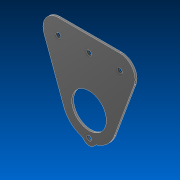
# Autodesk Inventor part: Intake Motor Holder Using 1__16 Gray Tinted Polycarbonate Sheet (36 x 72) (217-6627)
Saved by Autodesk Inventor 2022.2 (Build 262287000, 287)
## iProperties
Created: 2022-01-11
Part Number: Intake Motor Holder Using 1__16 Gray Tinted Polycarbonate Sheet (36 x 72) (217-6627)
Material: Polycarbonate, Clear
Document SubType Name: Modeling
Designer: omard
Density: 1.2 g/cm^3
Appearance: Smooth - Black
Author: omard
Autodesk Inventor part; units mm, degrees
ref_plane "YZ Plane" through (0, 0, 0) normal (1, 0, 0) x (0, 1, 0)
ref_plane "XZ Plane" through (0, 0, 0) normal (0, 1, 0) x (-1, 0, 0)
ref_plane "XY Plane" through (0, 0, 0) normal (0, 0, 1) x (1, 0, 0)
sketch "Sketch1" plane through (0, 0, 0) normal (0, 0, 1) x (1, 0, 0)
  circle A0 centre (0, 0) radius 14.2875
  circle A1 centre (-25.4, 41.275) radius 2.0701
  circle A2 centre (0, 41.275) radius 2.0701
  circle A3 centre (25.4, 41.275) radius 2.0701
  line L0 (-25.4, 41.275) -> (25.4, 41.275) construction
  circle A4 centre (0, 0) radius 22.225
  line L1 (-25.4, 41.275) -> (25.4, 41.275) construction
  line L2 (-25.4, 28.575) -> (25.4, 28.575) construction
  line L3 (25.4, 53.975) -> (-25.4, 53.975)
  arc A5 (-25.4, 53.975) -> (-25.4, 28.575) centre (-25.4, 41.275) ccw
  arc A6 (25.4, 28.575) -> (25.4, 53.975) centre (25.4, 41.275) ccw
  line L4 (-20.8482, -7.7008) -> (-37.3133, 36.8745)
  line L5 (1.8331, -22.86) -> (-1.8331, -22.86) construction
  line L6 (-1.8331, -22.86) -> (-3.6662, -19.685) construction
  line L7 (-3.6662, -19.685) -> (-1.8331, -16.51) construction
  line L8 (-1.8331, -16.51) -> (1.8331, -16.51) construction
  line L9 (1.8331, -16.51) -> (3.6662, -19.685) construction
  line L10 (3.6662, -19.685) -> (1.8331, -22.86) construction
  circle A7 centre (0, 0) radius 16.51 construction
  circle A8 centre (0, -19.685) radius 2.0701
  line L11 (0, -19.685) -> (0, 0) construction
  circle A9 centre (0, -19.685) radius 5.3975
  arc A10 (-4.2797, -22.9739) -> (-6.8869, -21.1311) centre (-8.5594, -26.2629) ccw
  arc A11 (6.8869, -21.1311) -> (4.2797, -22.9739) centre (8.5594, -26.2629) ccw
  circle A12 centre (0, -19.685) radius 4.0005 construction
  line L12 (20.8482, -7.7008) -> (37.3133, 36.8745)
  point P0 (0, -22.86)
  dimension "d0" = 25.4
  dimension "d4" = 4.1402
  dimension "d5" = 28.575
  dimension "d6" = 44.45
  dimension "d7" = 25.4
  dimension "d10" = 6.35
  dimension "d11" = 33.02
  dimension "d12" = 8.001
  dimension "d13" = 41.275
  constraints: 28 end point, 16 point on circle, 14 tangent, 13 centre point, 6 coincident, 5 equal radius, 3 midpoint, 2 equal length, 1 horizontal, 1 perpendicular, 1 point on line, 1 vertical alignment, 13 other
  measures "d0" distance of A2.centre L0.start
  measures "d4" diameter of A1
  measures "d5" diameter of A0
  measures "d6" diameter of A4
  measures "d7" diameter of A6
  measures "d10" distance from line of point (0, -22.86) L8
  measures "d11" diameter of A7
  measures "d12" diameter of A12
  measures "d13" distance of point (0, 0) A2.centre
extrude "Extrusion1" add sketch "Sketch1" along normal blind 1.5875
body "Solid1"
